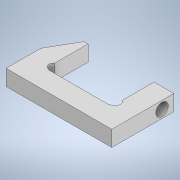
# Autodesk Inventor part: Practica 9
Saved by Autodesk Inventor 2020 (Build 240168000, 168)
## iProperties
Created: 2020-02-22
Part Number: Practica 9
Material: Genérico
Document SubType Name: Chapa
Designer: luisg
Density: 1 g/cm^3
Sheet Metal Rule: Por defecto_mm
Appearance: Valor por defecto
Author: luisg
Autodesk Inventor part; units mm, degrees
ref_plane "YZ Plane" through (0, 0, 0) normal (1, 0, 0) x (0, 1, 0)
ref_plane "XZ Plane" through (0, 0, 0) normal (0, 1, 0) x (-1, 0, 0)
ref_plane "XY Plane" through (0, 0, 0) normal (0, 0, 1) x (1, 0, 0)
sketch "Boceto1" plane through (0, 0, 0) normal (0, 1, 0) x (-1, 0, 0)
  line L0 (0, 0) -> (-80, 0)
  line L1 (-80, 0) -> (-80, -47)
  line L2 (-80, -47) -> (-65, -47)
  arc A0 (-63, -15.536) -> (-65, -23.0001) centre (-63, -19.536) ccw
  line L3 (0, 0) -> (-28.6172, 0) construction
  arc A1 (-15, -21.8283) -> (-17, -15.536) centre (-17, -19) ccw
  line L4 (0, 0) -> (-17, 0) construction
  line L5 (-65, -47) -> (-65, -23.0001)
  line L6 (-15, -47) -> (-12, -47)
  line L7 (-12, -47) -> (0, -26.2154)
  line L8 (0, -26.2154) -> (0, 0)
  line L9 (-15, -47) -> (-15, -21.8283)
  line L10 (-17, -15.536) -> (-17, -15)
  line L11 (-17, -15) -> (-63, -15)
  line L12 (-63, -15) -> (-63, -15.536)
  dimension "d0" = 80
  dimension "d1" = 47
  dimension "d2" = 15
  dimension "d6" = 8
  dimension "d7" = 17
  dimension "d8" = 3
  dimension "d9" = 15
  dimension "d10" = 30
  dimension "d11" = 19
  dimension "d14" = 17
  dimension "d15" = 17
  dimension "d16" = 47
  dimension "d17" = 15
  constraints: 26 end point, 4 perpendicular, 4 point on circle, 3 horizontal, 3 vertical, 2 centre point, 2 point on line
  measures "d0" distance of L0.start L0.end
  measures "d1" distance of L0.end L1.end
  measures "d2" distance of L1.end L2.end
  measures "d6" diameter of A0
  measures "d7" distance of L0.start L4.end
  measures "d8" distance of L6.start L6.end
  measures "d9" distance from line of L6.start L8
  measures "d10" angle of L9 L7
  measures "d11" distance from line of L0 A1.centre
  measures "d14" distance from line of L1 A0.centre
  measures "d15" distance from line of L8 A1.centre
  measures "d16" distance between parallel lines of L3 L6
  measures "d17" distance between parallel lines of L0 L11
extrude "Extrusión1" add sketch "Boceto1" along normal blind 12
sketch "Boceto2" plane through (80, 0, 0) normal (1, 0, 0) x (0, 0, -1)
  line L0 (26.2154, 12) -> (0, 12) construction
  line L1 (0, 12) -> (0, 6) construction
  line L2 (0, 0) -> (0, 12) construction
  line L3 (0, 6) -> (47, 6) construction
  line L4 (47, 0) -> (47, 12) construction
  circle A0 centre (38, 6) radius 4.75
  dimension "d22" = 9.5
  dimension "d23" = 38
  constraints: 4 end point, 2 midpoint, 1 centre point, 1 point on line
  measures "d22" diameter of A0
  measures "d23" distance from line of L2 A0.centre
extrude "Extrusión2" cut sketch "Boceto2" against normal up to surface (15 mm away)
equation "\"Radio_pliegue\" = Grosor"
equation "\"Anchura_desahogo_plegado\" = Grosor"
equation "\"Profundidad_desahogo_plegado\" = 0.5 * Grosor"
equation "\"Tamaño_destalonado\" = 4 * Grosor"
equation "\"Remanente_mínimo\" = 2 * Grosor"
equation "\"Radiodetransición\" = Radio_pliegue"
equation "\"Tamaño_de_radio_de_Jacobi\" = Radio_pliegue"
equation "\"TamañoSeparación\" = Grosor"
equation "\"Grosor\" = 0.5"
